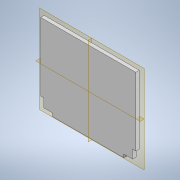
# Autodesk Inventor part: Side_Side_MDF
Saved by Autodesk Inventor 2021 (Build 250183000, 183)
## iProperties
Created: 2021-02-17
Part Number: Side_Side_MDF
Material: Generic
Document SubType Name: Modeling
Designer: negt20
Density: 1 g/cm^3
Appearance: Default
Author: negt20
Autodesk Inventor part; units mm, degrees
sketch "Sketch1" plane through (0, 0, 0) normal (0, 0, 1) x (1, 0, 0)
  line L0 (-80.5, 67.75) -> (80.5, 67.75)
  line L1 (80.5, 67.75) -> (80.5, -67.75)
  line L2 (80.5, -67.75) -> (-80.5, -67.75)
  line L3 (-80.5, -67.75) -> (-80.5, 67.75)
  point P0 (0, 67.75)
  point P1 (0, 0)
  point P2 (-80.5, 0)
  dimension "d0" = 161
  dimension "d1" = 135.5
  constraints: 8 end point, 2 midpoint, 2 parallel, 1 horizontal, 1 horizontal alignment, 1 perpendicular, 1 vertical alignment
  measures "d0" distance of L1.end L2.end
  measures "d1" distance of L0.end L1.end
extrude "Extrusion1" add sketch "Sketch1" along normal blind 6
sketch "Sketch2" plane through (0, 0, 6) normal (0, 0, 1) x (1, 0, 0)
  line L0 (-80.5, 67.75) -> (-80.5, -67.75) projected
  line L1 (-80.5, -67.75) -> (-80.5, -47.75)
  line L2 (-80.5, -47.75) -> (-75, -47.75)
  line L3 (-75, -47.75) -> (-75, -62.25)
  line L4 (-75, -62.25) -> (-60.5, -62.25)
  line L5 (-60.5, -62.25) -> (-60.5, -67.75)
  line L6 (-80.5, -67.75) -> (80.5, -67.75) projected
  line L7 (-60.5, -67.75) -> (-80.5, -67.75)
  point P0 (0, 0)
  point P1 (40.5, -62.5)
  dimension "d14" = 20
  dimension "d15" = 5.5
  dimension "d16" = 14.5
  dimension "d17" = 14.5
  constraints: 12 end point, 5 perpendicular, 1 point on line, 2 other
  measures "d14" distance of L0.end L1.end
  measures "d15" distance of L1.end L2.end
  measures "d16" distance of L2.end L3.end
  measures "d17" distance of L3.end L4.end
extrude "Extrusion2" cut sketch "Sketch2" against normal blind 15
mirror "Mirror1" about plane through (0, 0, 0) normal (1, 0, 0) of "Extrusion2"
equation "\"d7\" = d5"
equation "\"d5\" = 15"
body "Solid1"
